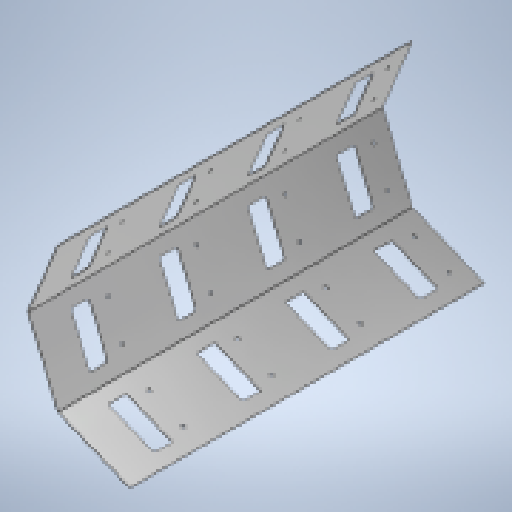
# Autodesk Inventor part: DMF 01 13 Барабан Лист лев брт v2.1
Saved by Autodesk Inventor 2025.4 (Build 294407000, 407)
## iProperties
Created: 2024-04-28
Part Number: DMF 01 13 Барабан Лист лев брт v2.1
Material: Stainless Steel AISI 304
Document SubType Name: Sheet Metal
Designer: pokla
Density: 8 g/cm^3
Appearance: Chrome - Satin
Sheet Metal Rule: Default
Flat Pattern Width: 63.3571 cm
Flat Pattern Length: 96 cm
Flat Pattern Area: 6082.28 cm^2
Sheet Metal Width: 633,571 mm
Sheet Metal Length: 960,000 mm
Sheet Metal Area: 608228,303 mm^2
Stock Number: Барабан_Лист_Левый_Борт
Author: pokla
Autodesk Inventor part; units mm, degrees
ref_plane "YZ Plane" through (0, 0, 0) normal (1, 0, 0) x (0, 1, 0)
ref_plane "XZ Plane" through (0, 0, 0) normal (0, 1, 0) x (-1, 0, 0)
ref_plane "XY Plane" through (0, 0, 0) normal (0, 0, 1) x (1, 0, 0)
sketch "Sketch2" plane through (0, 0, 0) normal (0, 0, 1) x (1, 0, 0)
  line L0 (0, 277.6336) -> (196.3166, 196.3166) construction
  line L1 (196.3166, 196.3166) -> (277.6336, 0) construction
  line L2 (277.6336, 0) -> (196.3166, -196.3166) construction
  line L3 (196.3166, -196.3166) -> (0, -277.6336) construction
  line L4 (0, -277.6336) -> (-196.3166, -196.3166) construction
  line L5 (-196.3166, -196.3166) -> (-277.6336, 0) construction
  line L6 (-277.6336, 0) -> (-196.3166, 196.3166) construction
  line L7 (-196.3166, 196.3166) -> (0, 277.6336) construction
  line L8 (-276.9995, -1.5307) -> (-196.9507, -194.7859)
  line L9 (-194.7859, -196.9507) -> (-0.8315, -277.2892)
  arc A0 (-276.9995, 1.5307) -> (-276.9995, -1.5307) centre (-273.304, 0) ccw
  arc A1 (-196.9507, -194.7859) -> (-194.7859, -196.9507) centre (-193.2551, -193.2551) ccw
  line L10 (-276.9995, 1.5307) -> (-196.661, 195.4851)
  point P0 (0, 0)
  point P1 (0, 0)
  dimension "d58" = 4
  dimension "d59" = 4
  dimension "d70" = 0.9
  dimension "d72" = 0.9
  dimension "d74" = 513
  measures "d58" radius of A0
  measures "d59" radius of A1
  measures "d70" distance of L3.end L9.end
  measures "d72" distance of L6.end L10.end
  measures "d74" distance between parallel lines of L1 L8
contour flange "Contour Flange3" sketch "Sketch2" thickness 2 bend radius 2 width 960 along (0, 0, -1) mid plane no both sides no wall seen from (-97.8087, -237.1199, 0) lies toward (0.3826834, 0.9238795, 0) curves L9 A1 L8 A0 L10
bend "Bend6"
corner "Corner6"
sketch "Sketch15" plane through (-276.9995, -1.5307, -960) normal (-0.9238795, -0.3826834, 0) x (0, 0, 1)
  line L0 (810, -37.0889) -> (860, -37.0889)
  line L1 (860, -37.0889) -> (860, -172.0889)
  line L2 (860, -172.0889) -> (810, -172.0889)
  line L3 (810, -172.0889) -> (810, -37.0889)
  circle A0 centre (765, -54.5889) radius 4.5
  circle A1 centre (765, -154.5889) radius 4.5
  line L4 (860, -104.5889) -> (810, -104.5889) construction
  line L5 (0, -209.1778) -> (0, 0) projected
  line L6 (960, -209.1778) -> (960, 0) projected
  point P0 (0, -104.5889)
  dimension "d192" = 9
  dimension "d193" = 135
  dimension "d194" = 50
  dimension "d195" = 45
  dimension "d196" = 100
  dimension "d207" = 100
  constraints: 10 end point, 3 midpoint, 2 centre point, 2 parallel, 1 horizontal, 1 horizontal alignment, 1 perpendicular, 1 other
  measures "d192" diameter of A0
  measures "d193" distance of L2.end L0.start
  measures "d194" distance of L0.start L0.end
  measures "d195" distance from line of A0.centre L3
  measures "d196" distance of A1.centre A0.centre
  measures "d207" distance between parallel lines of L6 L1
extrude "Cut1" cut sketch "Sketch15" against normal through all
fillet "Fillet2" radius 5 4 edges at (-210.2201, -160.1375, -150) (-210.2201, -160.1375, -100) (-261.8824, -35.4137, -100) (-261.8824, -35.4137, -150)
pattern_linear "Rectangular Pattern3" count 4 spacing 240 along (0, 0, -1) of "Cut1", "Fillet2"
pattern_circular "Circular Pattern3" count 3 over 90 about axis through (0, 0, -10) along (0, 0, 1) of "Cut1", "Rectangular Pattern3", "Fillet2" both ways yes
equation "\"d58\" = BendRadius + Thickness"
equation "\"d59\" = BendRadius + Thickness"
equation "\"d74\" = Барабан_габарит_по_кассетам"
equation "\"d75\" = Thickness"
equation "\"d76\" = BendReliefWidth"
equation "\"d77\" = BendReliefDepth"
equation "\"d78\" = MinimumRemnant"
equation "\"d79\" = TransitionRadius"
equation "\"d81\" = BendRadius"
equation "\"d83\" = CornerReliefSize"
equation "\"d84\" = GapSize"
equation "\"d85\" = JacobiRadiusSize"
equation "\"BendRadius\" = Thickness"
equation "\"BendReliefWidth\" = Thickness"
equation "\"BendReliefDepth\" = 0.5 * Thickness"
equation "\"CornerReliefSize\" = 4 * Thickness"
equation "\"MinimumRemnant\" = 2 * Thickness"
equation "\"TransitionRadius\" = BendRadius"
equation "\"JacobiRadiusSize\" = BendRadius"
equation "\"GapSize\" = Thickness"
equation "\"Барабан_Середина_листа\" = 206.27835"
equation "\"Thickness\" = 2"
equation "\"Барабан_габарит_по_кассетам\" = 513"
body "Solid3"
